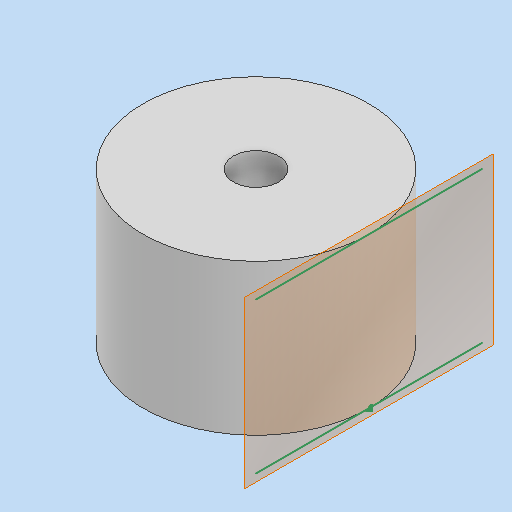
# Autodesk Inventor part: 微型联轴器
Saved by Autodesk Inventor 2026.2 (Build 302298010, 298A)
## iProperties
Created: 2026-03-17
Part Number: 微型联轴器
Material: 常规
Document SubType Name: Modeling
Designer: liu
Density: 1 g/cm^3
Appearance: 默认
Author: liu
Autodesk Inventor part; units mm, degrees
ref_plane "XZ Plane" through (0, 0, 0) normal (0, 1, 0) x (-1, 0, 0)
ref_plane "XY Plane" through (0, 0, 0) normal (0, 0, 1) x (1, 0, 0)
sketch "草图1" plane through (0, 0, 0) normal (0, 1, 0) x (-1, 0, 0)
  circle A0 centre (0, 0) radius 7.5
  dimension "d0" = 15
  constraints: 1 centre point, 1 coincident
  measures "d0" diameter of A0
extrude "拉伸1" add sketch "草图1" along normal blind 10
sketch "草图2" plane through (0, 10, 0) normal (0, 1, 0) x (1, 0, 0)
  circle A0 centre (0, 0) radius 1.5
  circle A1 centre (0, 0) radius 7.5 projected
  dimension "d3" = 3
  dimension "d4" = 0
  dimension "d5" = 0
  constraints: 1 centre point
  measures "d3" diameter of A0
  measures "d4" distance of A1.centre A0.centre
  measures "d5" distance of A1.centre A0.centre
extrude "拉伸2" cut sketch "草图2" against normal blind 10 contours A0
sketch "草图3" plane through (0, 0, 0) normal (0, -1, 0) x (1, 0, 0)
  point P0 (0, 0)
ref_plane "工作平面1" through (7.5, 0, 0) normal (1, 0, 0) x (0, 1, 0)
sketch "草图4" plane through (7.5, 0, 0) normal (1, 0, 0) x (0, 1, 0)
  line L0 (10, -7.5) -> (10, 7.5) projected
  line L1 (0, -7.5) -> (0, 7.5) projected
  point P0 (0, 0)
